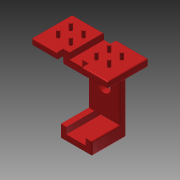
# Autodesk Inventor part: Spool Holder Main Section Mk1
Saved by Autodesk Inventor 2015 (Build 190159000, 159)
## iProperties
Created: 2016-11-23
Part Number: Spool Holder Main Section Mk1
Material: Generic
Document SubType Name: Modeling
Designer: Markus
Density: 1 g/cm^3
Appearance: Light Red
Author: Markus
Autodesk Inventor part; units mm, degrees
ref_plane "YZ Plane" through (0, 0, 0) normal (1, 0, 0) x (0, 1, 0)
ref_plane "XZ Plane" through (0, 0, 0) normal (0, 1, 0) x (-1, 0, 0)
ref_plane "XY Plane" through (0, 0, 0) normal (0, 0, 1) x (1, 0, 0)
sketch "Sketch1" plane through (0, 0, 0) normal (0, 0, 1) x (1, 0, 0)
  line L0 (0, 0) -> (76.2, 0)
  line L1 (76.2, 0) -> (76.2, -6.35)
  line L2 (76.2, -6.35) -> (0, -6.35)
  line L3 (0, -6.35) -> (0, 0)
  line L4 (0, -6.35) -> (22.225, -28.575)
  line L5 (76.2, -6.35) -> (53.975, -28.575)
  line L6 (22.225, -28.575) -> (22.225, -78.8162)
  line L7 (53.975, -28.575) -> (53.975, -78.8162)
  circle A0 centre (38.1, -39.37) radius 6.3881
  line L8 (31.6738, 0) -> (31.6738, -6.35)
  line L9 (44.5262, -6.35) -> (44.5262, 0)
  line L10 (25.3238, -6.35) -> (50.8762, -6.35)
  line L11 (50.8762, -6.35) -> (50.8762, -12.7)
  line L12 (50.8762, -12.7) -> (25.3238, -12.7)
  line L13 (25.3238, -12.7) -> (25.3238, -6.35)
  circle A1 centre (38.1, -39.37) radius 26.67 construction
  line L14 (28.4988, -66.04) -> (47.7012, -66.04)
  line L15 (47.7012, -66.04) -> (47.7012, -72.4662)
  line L16 (47.7012, -72.4662) -> (28.4988, -72.4662)
  line L17 (28.4988, -72.4662) -> (28.4988, -66.04)
  line L18 (22.225, -78.8162) -> (53.975, -78.8162)
  circle A2 centre (38.1, -39.37) radius 25.4 construction
  line L19 (38.1, -66.04) -> (38.1, -69.2531) construction
  line L20 (38.1, -69.2531) -> (47.7012, -69.2531) construction
  point P0 (38.1, 0)
  dimension "d0" = 76.2
  dimension "d1" = 6.35
  dimension "d2" = 45
  dimension "d3" = 45
  dimension "d4" = 31.75
  dimension "d6" = 12.7762
  dimension "d11" = 6.35
  dimension "d12" = 6.35
  dimension "d13" = 6.35
  dimension "d14" = 53.34
  dimension "d15" = 6.2738
  dimension "d16" = 6.2738
  dimension "d17" = 6.35
  dimension "d18" = 6.4262
  dimension "d19" = 6.4262
  dimension "d20" = 6.4262
  dimension "d21" = 50.8
  dimension "d40" = 69.2531
  dimension "d41" = 19.2024
  dimension "d42" = 39.37
  constraints: 42 end point, 7 parallel, 5 horizontal, 5 point on line, 4 perpendicular, 3 centre point, 3 midpoint, 3 vertical, 2 coincident, 2 horizontal alignment, 2 tangent, 1 vertical alignment
  measures "d0" distance of L0.start L0.end
  measures "d1" distance of L2.end L0.start
  measures "d2" angle of L4 L2
  measures "d3" angle of L5 L2
  measures "d4" distance between parallel lines of L7 L6
  measures "d6" diameter of A0
  measures "d11" distance between parallel lines of L8 L13
  measures "d12" distance between parallel lines of L9 L11
  measures "d13" distance between parallel lines of L10 L12
  measures "d14" diameter of A1
  measures "d15" distance between parallel lines of L17 L6
  measures "d16" distance between parallel lines of L7 L15
  measures "d17" distance between parallel lines of L18 L16
  measures "d18" distance between parallel lines of L16 L14
  measures "d19" distance from line of A0.centre L8
  measures "d20" distance from line of L9 A1.centre
  measures "d21" diameter of A2
  measures "d40" distance from line of L20.end L0
  measures "d41" distance between parallel lines of L15 L17
  measures "d42" distance from line of L0 A0.centre
extrude "Extrusion1" add sketch "Sketch1" along normal blind 6.35 contours L0 L8 L2 L3 | L2 L13 L12 L11 L5 L7 L18 L6 L4 | L0 L1 L2 L9 | L2 L11 L12 L13
sketch "Sketch3" plane through (0, 0, 6.35) normal (0, 0, 1) x (1, 0, 0)
  line L0 (0, 0) -> (31.6738, 0)
  line L1 (31.6738, 0) -> (31.6738, -6.35)
  line L2 (31.6738, -6.35) -> (0, -6.35)
  line L3 (0, -6.35) -> (0, 0)
  line L4 (44.5262, -6.35) -> (76.2, -6.35)
  line L5 (76.2, -6.35) -> (76.2, 0)
  line L6 (76.2, 0) -> (44.5262, 0)
  line L7 (44.5262, 0) -> (44.5262, -6.35)
  line L8 (50.8762, -6.35) -> (25.3238, -6.35)
  line L9 (25.3238, -6.35) -> (25.3238, -12.7)
  line L10 (25.3238, -12.7) -> (50.8762, -12.7)
  line L11 (50.8762, -12.7) -> (50.8762, -6.35)
  line L12 (22.225, -28.575) -> (22.225, -78.8162) projected
  line L13 (28.4988, -66.04) -> (22.225, -66.04)
  line L14 (22.225, -66.04) -> (22.225, -72.4662)
  line L15 (22.225, -72.4662) -> (28.4988, -72.4662)
  line L16 (28.4988, -72.4662) -> (28.4988, -66.04)
  line L17 (53.975, -78.8162) -> (53.975, -28.575) projected
  line L18 (22.225, -78.8162) -> (53.975, -78.8162)
  line L19 (53.975, -78.8162) -> (53.975, -72.4662)
  line L20 (53.975, -72.4662) -> (22.225, -72.4662)
  line L21 (22.225, -72.4662) -> (22.225, -78.8162)
  line L22 (47.7012, -66.04) -> (53.975, -66.04)
  line L23 (53.975, -66.04) -> (53.975, -72.4662)
  line L24 (53.975, -72.4662) -> (47.7012, -72.4662)
  line L25 (47.7012, -72.4662) -> (47.7012, -66.04)
  dimension "d22" = 6.35
  dimension "d23" = 6.35
  dimension "d24" = 6.35
  constraints: 48 end point, 12 parallel, 6 horizontal, 6 perpendicular, 6 point on line, 2 coincident, 1 horizontal alignment
  measures "d22" distance between parallel lines of L1 L9
  measures "d23" distance between parallel lines of L7 L11
  measures "d24" distance between parallel lines of L8 L10
extrude "Extrusion2" add sketch "Sketch3" along normal blind 27.94
sketch "Sketch4" plane through (0, 0, 34.29) normal (0, 0, 1) x (1, 0, 0)
  line L0 (44.5262, -6.35) -> (31.6738, -6.35) projected
  line L1 (31.6738, -6.35) -> (31.6738, 0) projected
  line L2 (31.6738, 0) -> (0, 0) projected
  line L3 (0, 0) -> (0, -6.35) projected
  line L4 (0, -6.35) -> (25.3238, -6.35) projected
  line L5 (25.3238, -6.35) -> (25.3238, -12.7) projected
  line L6 (25.3238, -12.7) -> (50.8762, -12.7) projected
  line L7 (50.8762, -12.7) -> (50.8762, -6.35) projected
  line L8 (50.8762, -6.35) -> (76.2, -6.35) projected
  line L9 (76.2, -6.35) -> (76.2, 0) projected
  line L10 (76.2, 0) -> (44.5262, 0) projected
  line L11 (44.5262, 0) -> (44.5262, -6.35) projected
  line L12 (53.975, -66.04) -> (47.7012, -66.04) projected
  line L13 (47.7012, -66.04) -> (47.7012, -72.4662) projected
  line L14 (47.7012, -72.4662) -> (28.4988, -72.4662) projected
  line L15 (28.4988, -72.4662) -> (28.4988, -66.04) projected
  line L16 (28.4988, -66.04) -> (22.225, -66.04) projected
  line L17 (22.225, -66.04) -> (22.225, -78.8162) projected
  line L18 (22.225, -78.8162) -> (53.975, -78.8162) projected
  line L19 (53.975, -78.8162) -> (53.975, -66.04) projected
  line L20 (0, 0) -> (25.3238, 0)
  line L21 (25.3238, 0) -> (25.3238, -6.35)
  line L22 (25.3238, -6.35) -> (0, -6.35)
  line L23 (0, -6.35) -> (0, 0)
  line L24 (50.8762, -6.35) -> (76.2, -6.35)
  line L25 (76.2, -6.35) -> (76.2, 0)
  line L26 (76.2, 0) -> (50.8762, 0)
  line L27 (50.8762, 0) -> (50.8762, -6.35)
  line L28 (22.225, -66.04) -> (28.4988, -66.04)
  line L29 (28.4988, -66.04) -> (28.4988, -72.4662)
  line L30 (28.4988, -72.4662) -> (47.7012, -72.4662)
  line L31 (47.7012, -72.4662) -> (47.7012, -66.04)
  line L32 (47.7012, -66.04) -> (53.975, -66.04)
  line L33 (53.975, -66.04) -> (53.975, -78.8162)
  line L34 (53.975, -78.8162) -> (22.225, -78.8162)
  line L35 (22.225, -78.8162) -> (22.225, -66.04)
  constraints: 32 end point, 6 equal length, 5 perpendicular, 4 horizontal
extrude "Extrusion3" add sketch "Sketch4" along normal blind 6.35 contours L10 L9 L8 L27 | L21 L4 L3 L2
sketch "Sketch5" plane through (0, 0, 0) normal (0, 1, 0) x (1, 0, 0)
  line L0 (31.6738, 0) -> (0, 0) projected
  line L1 (0, 0) -> (0, -40.64) projected
  line L2 (25.3238, -40.64) -> (0, -40.64) projected
  line L3 (25.3238, -34.29) -> (25.3238, -40.64) projected
  line L4 (31.6738, -34.29) -> (25.3238, -34.29) projected
  line L5 (31.6738, 0) -> (31.6738, -34.29) projected
  line L6 (76.2, 0) -> (44.5262, 0) projected
  line L7 (44.5262, 0) -> (44.5262, -34.29) projected
  line L8 (50.8762, -34.29) -> (44.5262, -34.29) projected
  line L9 (50.8762, -34.29) -> (50.8762, -40.64) projected
  line L10 (76.2, -40.64) -> (50.8762, -40.64) projected
  line L11 (76.2, 0) -> (76.2, -40.64) projected
  line L12 (44.5262, 0) -> (31.6738, 0) projected
  line L13 (0, 0) -> (76.2, -40.64) construction
  line L14 (76.2, 0) -> (0, -40.64) construction
  line L15 (38.1, -20.32) -> (0, -20.32) construction
  circle A0 centre (25.4, -13.97) radius 1.5875
  circle A1 centre (25.4, -26.67) radius 1.5875
  circle A2 centre (12.7, -13.97) radius 1.5875
  circle A3 centre (12.7, -26.67) radius 1.5875
  circle A4 centre (50.8, -13.97) radius 1.5875
  circle A5 centre (50.8, -26.67) radius 1.5875
  circle A6 centre (63.5, -13.97) radius 1.5875
  circle A7 centre (63.5, -26.67) radius 1.5875
  line L16 (63.5, -13.97) -> (12.7, -26.67) construction
  line L17 (12.7, -26.67) -> (63.5, -26.67) construction
  line L18 (63.5, -26.67) -> (12.7, -13.97) construction
  line L19 (12.7, -13.97) -> (63.5, -13.97) construction
  dimension "d29" = 3.175
  dimension "d31" = 6.35
  dimension "d32" = 12.7
  dimension "d33" = 6.35
  dimension "d34" = 25.4
  dimension "d35" = 12.7
  dimension "d37" = 25.4
  constraints: 14 end point, 8 centre point, 7 equal radius, 6 horizontal alignment, 4 vertical alignment, 2 midpoint, 1 horizontal, 1 parallel
  measures "d29" diameter of A0
  measures "d31" distance from line of L15 A0.centre
  measures "d32" horizontal distance of L15.start A0.centre
  measures "d33" distance from line of L15 A1.centre
  measures "d34" horizontal distance of L15.start L18.end
  measures "d35" horizontal distance of A4.centre L15.start
  measures "d37" horizontal distance of L16.start L15.start
extrude "Extrusion4" add sketch "Sketch5" along normal blind 6.35 contours A0 | A1 | A2 | A3 | A4 | A5 | A6 | A7
fillet "Fillet1" radius 1.27 36 edges at (12.6619, 0, 40.64) (12.6619, -6.35, 40.64) (63.5381, -6.35, 40.64) (63.5381, 0, 40.64) (76.2, -6.35, 23.495) (76.2, 0, 20.32) (76.2, -6.35, 3.175) (60.3631, 0, 0) (15.8369, 0, 0) (0, 0, 20.32) (0, -6.35, 23.495) (0, -6.35, 3.175) (11.1125, -17.4625, 6.35) (11.1125, -17.4625, 0) (22.225, -47.3075, 6.35) (22.225, -53.6956, 0) (65.0875, -17.4625, 6.35) (65.0875, -17.4625, 0) (53.975, -47.3075, 6.35) (53.975, -53.6956, 0) (53.975, -66.04, 20.32) (22.225, -66.04, 20.32) (22.225, -72.4281, 34.29) (38.1, -78.8162, 34.29) (53.975, -72.4281, 34.29) (53.975, -78.8162, 17.145) (22.225, -78.8162, 17.145) (38.1, -78.8162, 0) (25.3238, -12.7, 20.32) (50.8762, -12.7, 20.32) (25.3238, -6.35, 20.32) (50.8762, -6.35, 20.32) (76.2, -3.175, 40.64) (76.2, -3.175, 0) (0, -3.175, 0) (0, -3.175, 40.64)
equation "\"d16\" = d15"
equation "\"d20\" = d19"
equation "\"d33\" = d31"
equation "\"d35\" = d32"
equation "\"d37\" = d34"
body "Solid1"
